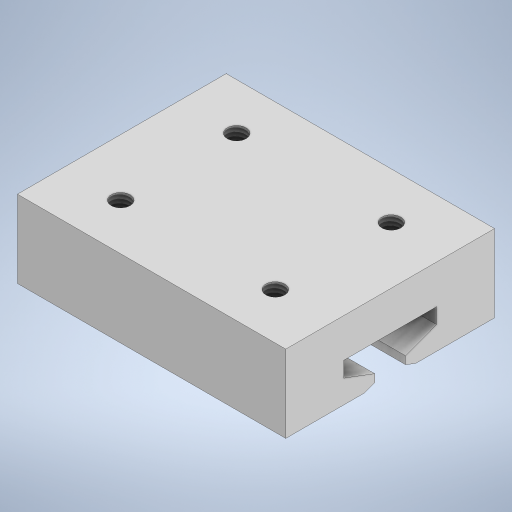
# Autodesk Inventor part: lm_guide_cart
Saved by Autodesk Inventor 2024 (Build 280153000, 153)
## iProperties
Created: 2023-09-15
Part Number: lm_guide_cart
Material: Generic
Document SubType Name: Modeling
Designer: 박동준
Density: 1 g/cm^3
Appearance: Default
Author: 박동준
Autodesk Inventor part; units mm, degrees
ref_plane "YZ Plane" through (0, 0, 0) normal (1, 0, 0) x (0, 1, 0)
ref_plane "XZ Plane" through (0, 0, 0) normal (0, 1, 0) x (-1, 0, 0)
ref_plane "XY Plane" through (0, 0, 0) normal (0, 0, 1) x (1, 0, 0)
sketch "Sketch1" plane through (0, 0, 0) normal (1, 0, 0) x (0, 1, 0)
  line L0 (5, 6) -> (3, 6)
  line L1 (3, 6) -> (1.5, 2)
  line L2 (1.5, 2) -> (0.5, 2)
  line L3 (0, 13.5) -> (10, 13.5)
  line L4 (10, 13.5) -> (10, 0)
  line L5 (5, 6) -> (5, 0)
  line L6 (10, 0) -> (-5, 0) construction
  line L7 (1.5, -2) -> (0.5, -2)
  line L8 (0.5, 2) -> (0, 3.3331)
  line L9 (0, 3.3331) -> (0, 13.5)
  line L10 (5, -6) -> (3, -6)
  line L11 (3, -6) -> (1.5, -2)
  line L12 (1.5, -2) -> (0.5, -2)
  line L13 (0, -13.5) -> (10, -13.5)
  line L14 (10, -13.5) -> (10, 0)
  line L15 (5, -6) -> (5, 0)
  line L16 (0.5, -2) -> (0, -3.3331)
  line L17 (0, -3.3331) -> (0, -13.5)
  point P0 (0, 0)
  point P1 (4, 6)
  point P2 (5, 13.5)
  point P3 (1, 2)
  point P4 (4, -6)
  dimension "d11" = 2
  dimension "d19" = 10
  dimension "d20" = 13.5
  dimension "d21" = 5
  dimension "d23" = 6
  dimension "d38" = 1
  dimension "d39" = 4
  dimension "d40" = 2
  dimension "d41" = 110.56
  constraints: 36 end point, 8 symmetric about line, 3 midpoint, 3 vertical, 2 horizontal alignment, 2 parallel, 1 horizontal, 1 vertical alignment
  measures "d11" distance of L0.start L0.end
  measures "d19" distance of L3.start L3.end
  measures "d20" distance of L3.end L4.end
  measures "d21" distance between parallel lines of L4 L5
  measures "d23" distance between parallel lines of L0 L6
  measures "d38" distance of L1.end L2.end
  measures "d39" distance from line of L5 point (1, 2)
  measures "d40" distance between parallel lines of L6 L2
  measures "d41" angle of L8 L2
extrude "Extrusion1" add sketch "Sketch1" along normal blind 34.7
sketch "Sketch2" plane through (0, 10, 13.5) normal (0, 1, 0) x (1, 0, 0)
  line L0 (0, 27) -> (0, 0) projected
  line L1 (0, 0) -> (34.7, 0) projected
  line L2 (34.7, 27) -> (34.7, 0) projected
  line L3 (0, 27) -> (34.7, 27) projected
  line L4 (7.35, 6) -> (7.35, 21) construction
  line L5 (7.35, 21) -> (27.35, 21) construction
  point P0 (0, 13.5)
  point P1 (27.35, 6)
  point P2 (7.35, 13.5)
  point P3 (0, 13.5)
  point P4 (17.35, 21)
  point P5 (17.35, 27)
  dimension "d29" = 20
  dimension "d30" = 15
  constraints: 4 end point, 4 midpoint, 2 horizontal alignment, 2 vertical alignment, 1 horizontal, 1 vertical
  measures "d29" distance of L4.end L5.end
  measures "d30" distance of L4.end L4.start
hole "Hole1" at (7.35, 10, 7.5) at (7.35, 10, -7.5) at (27.35, 10, -7.5) at (27.35, 10, 7.5) direction (0, -1, 0) diameter 2.459 depth 6 thread size "M3x0.5" class "6H" standard "ISO Metric profile"
body "Solid1"
